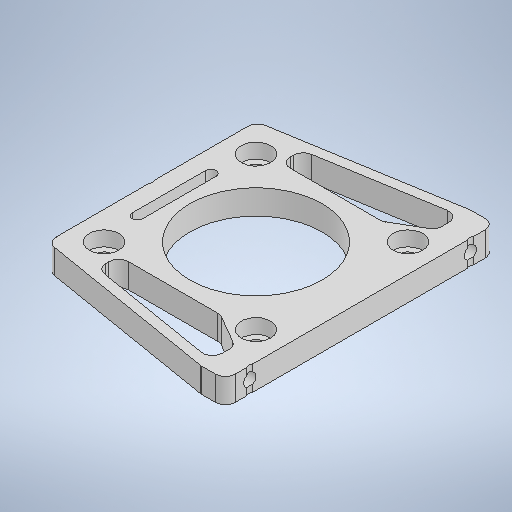
# Autodesk Inventor part: T5.0_stepper-fix
Saved by Autodesk Inventor 2025 (Build 290162000, 162)
## iProperties
Created: 2024-06-29
Part Number: T5.0_stepper-fix
Material: 一般
Document SubType Name: Sheet Metal
Designer: 8326d
Density: 1 g/cm^3
Sheet Metal Rule: Default_mm
Appearance: 既定
Author: 8326d
Autodesk Inventor part; units mm, degrees
ref_plane "YZ Plane" through (0, 0, 0) normal (1, 0, 0) x (0, 1, 0)
ref_plane "XZ Plane" through (0, 0, 0) normal (0, 1, 0) x (-1, 0, 0)
ref_plane "XY Plane" through (0, 0, 0) normal (0, 0, 1) x (1, 0, 0)
sketch "スケッチ1" plane through (0, 0, 0) normal (0, 1, 0) x (-1, 0, 0)
  line L0 (-21.25, 21.25) -> (21.25, 21.25)
  line L1 (21.25, 21.25) -> (21.25, -21.25)
  line L2 (21.25, -21.25) -> (-21.25, -21.25)
  line L3 (-21.25, -21.25) -> (-21.25, 21.25)
  line L4 (-21.25, 21.25) -> (21.25, -21.25) construction
  line L5 (21.25, 21.25) -> (-21.25, -21.25) construction
  line L6 (-21.25, 27.5) -> (-16.25, 27.5)
  line L7 (-16.25, 27.5) -> (-16.25, -27.5)
  line L8 (-16.25, -27.5) -> (-21.25, -27.5)
  line L9 (-21.25, -27.5) -> (-21.25, 27.5)
  line L10 (-21.25, 27.5) -> (-16.25, -27.5) construction
  line L11 (-16.25, 27.5) -> (-21.25, -27.5) construction
  line L12 (21.25, 21.25) -> (-16.25, 27.5)
  line L13 (-16.25, -27.5) -> (21.25, -21.25)
  point P0 (0, 0)
  point P1 (-18.75, 0)
  dimension "d0" = 42.5
  dimension "d1" = 42.5
  dimension "d12" = 6.25
  dimension "d13" = 5
  measures "d0" distance of L1.end L2.end
  measures "d1" distance of L0.end L1.end
  measures "d12" distance between parallel lines of L8 L2
  measures "d13" distance of L6.start L6.end
extrude "プレート1" add sketch "スケッチ1" along normal blind 5
sketch "スケッチ2" plane through (0, 5, 0) normal (0, 1, 0) x (1, 0, 0)
  line L0 (15.5, -15.5) -> (-15.5, -15.5) construction
  line L1 (-15.5, -15.5) -> (-15.5, 15.5) construction
  line L2 (-15.5, 15.5) -> (15.5, 15.5) construction
  line L3 (15.5, 15.5) -> (15.5, -15.5) construction
  line L4 (15.5, -15.5) -> (-15.5, 15.5) construction
  line L5 (-15.5, -15.5) -> (15.5, 15.5) construction
  point P0 (0, 0)
  dimension "d3" = 31
  dimension "d4" = 31
  constraints: 12 end point, 2 midpoint, 2 parallel, 1 horizontal, 1 perpendicular
  measures "d3" distance of L1.end L2.end
  measures "d4" distance of L0.end L1.end
hole "穴1" at (15.5, 5, 15.5) at (15.5, 5, -15.5) at (-15.5, 5, -15.5) at (-15.5, 5, 15.5) direction (0, -1, 0) diameter 3.5 depth 5 tip angle 118 counterbore diameter 6 counterbore depth 3
sketch "スケッチ3" plane through (0, 5, 0) normal (0, 1, 0) x (1, 0, 0)
  line L0 (21.25, 27.5) -> (21.25, -27.5) projected
  circle A0 centre (22.1, -22.5) radius 1.05
  line L1 (21.25, -27.5) -> (16.25, -27.5) projected
  line L2 (16.25, -27.5) -> (-21.25, -21.25) projected
  line L3 (-11.5, -20.8474) -> (16.25, -25.4724)
  line L4 (16.25, -25.4724) -> (16.25, -20.5518)
  line L5 (16.25, -20.5518) -> (9.2321, -16.5)
  line L6 (9.2321, -16.5) -> (-11.5, -16.5)
  line L7 (-11.5, -16.5) -> (-11.5, -20.8474)
  line L8 (-21.25, -21.25) -> (-21.25, 21.25) projected
  circle A1 centre (15.5, -15.5) radius 1.75 projected
  circle A2 centre (-15.5, -15.5) radius 1.75 projected
  point P0 (0, 0)
  dimension "d14" = 2.1
  dimension "d15" = 0.85
  dimension "d16" = 5
  dimension "d19" = 2
  dimension "d20" = 5
  dimension "d21" = 4
  dimension "d22" = 1
  dimension "d23" = 4
  dimension "d24" = 120
  constraints: 10 end point, 3 parallel, 3 perpendicular, 1 centre point, 1 vertical
  measures "d14" diameter of A0
  measures "d15" distance from line of L0 A0.centre
  measures "d16" distance from line of L1 A0.centre
  measures "d19" distance between parallel lines of L2 L3
  measures "d20" distance between parallel lines of L0 L4
  measures "d21" distance from line of A1.centre L5
  measures "d22" distance from line of A1.centre L6
  measures "d23" distance from line of A2.centre L7
  measures "d24" angle of L4 L5
extrude "押し出し1" cut sketch "スケッチ3" against normal through all contours A0 L0 | L0 A0 | L7 L6 L5 L4 L3
fillet "フィレット1" radius 2 5 edges at (16.25, 2.5, 25.4724) (16.25, 2.5, 20.5518) (9.2321, 2.5, 16.5) (-11.5, 2.5, 16.5) (-11.5, 2.5, 20.8474)
sketch "スケッチ4" plane through (21.25, 0, 27.5) normal (1, 0, 0) x (0, 0, -1)
  line L0 (4.3836, 0) -> (4.3836, 5) projected
  line L1 (5.6164, 0) -> (4.3836, 0) projected
  line L2 (5.6164, 5) -> (5.6164, 0) projected
  line L3 (4.3836, 5) -> (5.6164, 5) projected
  point P0 (27.5, 0)
  point P1 (5, 2.5)
  point P2 (5, 5)
  point P3 (4.3836, 2.5)
  constraints: 2 midpoint, 1 horizontal alignment, 1 vertical alignment
hole "穴2" at (21.25, 2.5, 22.5) direction (-1, 0, 0) diameter 2.5 depth 8 tip angle 118
mirror "ミラー1" about plane through (0, 0, 0) normal (0, 0, 1) of "押し出し1", "フィレット1", "穴2"
sketch "スケッチ5" plane through (0, 5, 0) normal (0, 1, 0) x (1, 0, 0)
  circle A0 centre (0, 0) radius 13.5
  dimension "d33" = 27
  constraints: 1 centre point, 1 coincident
  measures "d33" diameter of A0
extrude "押し出し2" cut sketch "スケッチ5" against normal through all
fillet "フィレット2" radius 2 6 edges at (-21.25, 2.5, 21.25) (-21.25, 2.5, -21.25) (16.25, 2.5, -27.5) (21.25, 2.5, -27.5) (21.25, 2.5, 27.5) (16.25, 2.5, 27.5)
sketch "スケッチ6" plane through (0, 5, 0) normal (0, 1, 0) x (1, 0, 0)
  line L0 (-21.25, -19.5557) -> (-21.25, 19.5557) projected
  circle A0 centre (-22.1, 0) radius 1.05
  point P0 (0, 0)
  dimension "d37" = 2.1
  dimension "d38" = 0.85
  constraints: 1 centre point, 1 horizontal alignment
  measures "d37" diameter of A0
  measures "d38" distance from line of L0 A0.centre
extrude "押し出し3" cut sketch "スケッチ6" against normal through all
sketch "スケッチ7" plane through (0, 5, 0) normal (0, 1, 0) x (1, 0, 0)
  line L0 (-16.7, -7.5) -> (-16.7, 7.5) construction
  line L1 (-15.65, -7.5) -> (-15.65, 7.5)
  line L2 (-17.75, 7.5) -> (-17.75, -7.5)
  arc A0 (-17.75, -7.5) -> (-15.65, -7.5) centre (-16.7, -7.5) ccw
  arc A1 (-15.65, 7.5) -> (-17.75, 7.5) centre (-16.7, 7.5) ccw
  line L3 (-21.25, 0.6164) -> (-21.25, 19.5557) projected
  point P0 (0, 0)
  point P1 (-16.7, 0)
  dimension "d41" = 3.5
  dimension "d42" = 2.1
  dimension "d43" = 15
  constraints: 8 end point, 4 point on circle, 4 tangent, 2 centre point, 1 horizontal alignment, 1 midpoint, 1 parallel, 1 vertical
  measures "d41" distance between parallel lines of L3 L2
  measures "d42" distance between parallel lines of L2 L1
  measures "d43" distance of L0.start L0.end
extrude "押し出し4" cut sketch "スケッチ7" against normal through all
equation "\"d10\" = Thickness"
equation "\"d23\" = d21"
equation "\"d2\" = Thickness"
equation "\"BendRadius\" = Thickness"
equation "\"BendReliefWidth\" = Thickness"
equation "\"BendReliefDepth\" = 0.5 * Thickness"
equation "\"TransitionRadius\" = BendRadius"
equation "\"JacobiRadiusSize\" = BendRadius"
equation "\"GapSize\" = Thickness"
equation "\"Thickness\" = 5"
